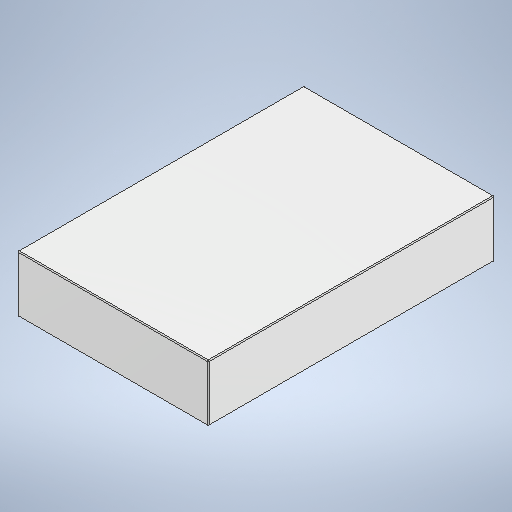
# Autodesk Inventor part: Part245
Saved by Autodesk Inventor 2025 (Build 290162000, 162)
## iProperties
Created: 2024-07-31
Part Number: Part245
Material: Generic
Document SubType Name: Modeling
Designer: Isaac
Density: 1 g/cm^3
Appearance: Default
Author: Isaac
Autodesk Inventor part; units mm, degrees
ref_plane "YZ Plane" through (0, 0, 0) normal (1, 0, 0) x (0, 1, 0)
ref_plane "XZ Plane" through (0, 0, 0) normal (0, 1, 0) x (-1, 0, 0)
ref_plane "XY Plane" through (0, 0, 0) normal (0, 0, 1) x (1, 0, 0)
sketch "Sketch1" plane through (0, 0, 0) normal (0, 0, 1) x (1, 0, 0)
  line L0 (-200, 119) -> (200, 119)
  line L1 (200, 119) -> (200, 0)
  line L2 (200, 0) -> (-200, 0)
  line L3 (-200, 0) -> (-200, 119)
  point P0 (0, 0)
  point P1 (0, 0)
  dimension "d0" = 119
  dimension "d1" = 400
  constraints: 8 end point, 2 parallel, 1 coincident, 1 horizontal, 1 midpoint, 1 perpendicular
  measures "d0" distance of L2.end L0.start
  measures "d1" distance of L0.start L0.end
extrude "Extrusion1" add sketch "Sketch1" along normal blind 600
fillet "Fillet1" radius 2 12 edges at (200, 119, 300) (0, 119, 600) (-200, 119, 300) (0, 119, 0) (200, 0, 300) (0, 0, 600) (200, 59.5, 600) (-200, 59.5, 600) (-200, 0, 300) (-200, 59.5, 0) (0, 0, 0) (200, 59.5, 0)
body "Solid1"
